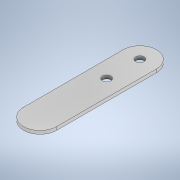
# Autodesk Inventor part: Sostenedores Contenedor
Saved by Autodesk Inventor 2020.3 (Build 243373000, 373)
## iProperties
Created: 2020-07-23
Part Number: Sostenedores Contenedor
Material: Generic
Document SubType Name: Modeling
Designer: juanp
Density: 1 g/cm^3
Appearance: Default
Author: juanp
Autodesk Inventor part; units mm, degrees
ref_plane "YZ Plane" through (0, 0, 0) normal (1, 0, 0) x (0, 1, 0)
ref_plane "XZ Plane" through (0, 0, 0) normal (0, 1, 0) x (-1, 0, 0)
ref_plane "XY Plane" through (0, 0, 0) normal (0, 0, 1) x (1, 0, 0)
sketch "Sketch1" plane through (0, 0, 0) normal (0, 1, 0) x (-1, 0, 0)
  line L0 (0, 0) -> (0, -80) construction
  line L1 (-10, -10) -> (-10, -70)
  line L2 (10, -70) -> (10, -10)
  arc A0 (10, -10) -> (-10, -10) centre (0, -10) ccw
  arc A1 (-10, -70) -> (10, -70) centre (0, -70) ccw
  circle A2 centre (0, -70) radius 2.55
  line L3 (0, -70) -> (0, -50) construction
  circle A3 centre (0, -50) radius 2.55
  point P0 (0, -40)
  dimension "d0" = 80
  dimension "d1" = 20
  dimension "d2" = 5.1
  dimension "d3" = 20
  dimension "d4" = 5.1
  constraints: 10 end point, 6 point on circle, 4 centre point, 4 tangent, 3 point on line, 2 coincident, 1 midpoint, 1 parallel, 1 vertical
  measures "d0" distance of L0.start L0.end
  measures "d1" diameter of A1
  measures "d2" diameter of A2
  measures "d3" distance of L3.start L3.end
  measures "d4" diameter of A3
extrude "Extrusion1" add sketch "Sketch1" along normal blind 2
body "Solid1"
